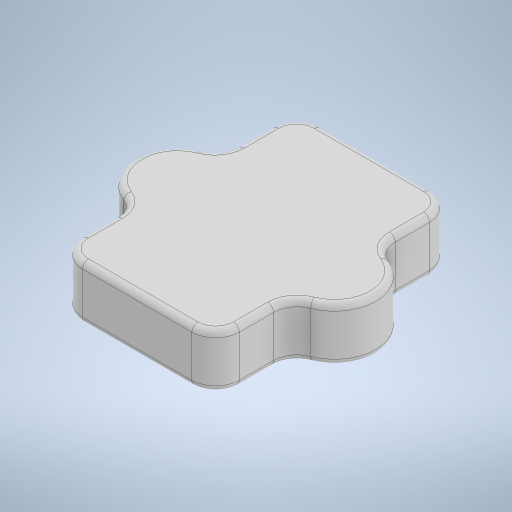
# Autodesk Inventor part: FuselageLock
Saved by Autodesk Inventor 2023 (Build 270158000, 158)
## iProperties
Created: 2023-11-15
Part Number: FuselageLock
Material: Generic
Document SubType Name: Modeling
Designer: Eric
Density: 1 g/cm^3
Appearance: Default
Author: Eric
Autodesk Inventor part; units mm, degrees
ref_plane "YZ Plane" through (0, 0, 0) normal (1, 0, 0) x (0, 1, 0)
ref_plane "XZ Plane" through (0, 0, 0) normal (0, 1, 0) x (-1, 0, 0)
ref_plane "XY Plane" through (0, 0, 0) normal (0, 0, 1) x (1, 0, 0)
sketch "Sketch1" plane through (0, 0, 0) normal (0, 1, 0) x (-1, 0, 0)
  line L0 (6.6, -10) -> (-6.6, -10)
  line L1 (-6.6, -10) -> (-6.6, 10)
  line L2 (-6.6, 10) -> (6.6, 10)
  line L3 (6.6, 10) -> (6.6, -10)
  point P0 (0, 0)
  point P1 (0, -10)
  point P2 (-6.6, 0)
  dimension "d0" = 13.2
  dimension "d1" = 20
  constraints: 8 end point, 2 midpoint, 2 parallel, 1 horizontal, 1 horizontal alignment, 1 perpendicular, 1 vertical alignment
  measures "d0" distance of L0.start L0.end
  measures "d1" distance of L0.end L1.end
extrude "Extrusion1" add sketch "Sketch1" along normal blind 4.5
sketch "Sketch2" plane through (0, 0, 0) normal (0, -1, 0) x (1, 0, 0)
  line L0 (6.6, 10) -> (6.6, -10) projected
  circle A0 centre (6.6, 0) radius 2
  line L1 (-6.6, -10) -> (-6.6, 10) projected
  circle A1 centre (-6.6, 0) radius 2
  circle A2 centre (6.6, 0) radius 3.5
  circle A3 centre (-6.6, 0) radius 3.5
  point P0 (0, 0)
  dimension "d4" = 4
  dimension "d5" = 7
  constraints: 4 centre point, 2 coincident, 2 equal radius, 2 midpoint
  measures "d4" diameter of A0
  measures "d5" diameter of A2
extrude "Extrusion2" add sketch "Sketch2" against normal blind 4.5
extrude "Extrusion3" cut sketch "Sketch2" against normal blind 3 contours A0 L0 | L0 A0 | A1 L1 | L1 A1
fillet "Fillet1" radius 2 8 edges at (6.6, 2.25, -10) (-6.6, 2.25, -10) (6.6, 2.25, 10) (-6.6, 2.25, 10) (6.6, 2.25, -3.5) (6.6, 2.25, 3.5) (-6.6, 2.25, -3.5) (-6.6, 2.25, 3.5)
fillet "Fillet2" radius 0.5 32 edges at (-6.9486, 0, -3.9953) (-6.6, 0, -6.5617) (-6.0142, 0, -9.4142) (0, 0, -10) (6.0142, 0, -9.4142) (6.6, 0, -6.5617) (6.9486, 0, -3.9953) (10.1, 0, 0) (6.9486, 0, 3.9953) (6.6, 0, 6.5617) (6.0142, 0, 9.4142) (0, 0, 10) (-6.0142, 0, 9.4142) (-6.6, 0, 6.5617) (-6.9486, 0, 3.9953) (-10.1, 0, 0) (-6.9486, 4.5, 3.9953) (-6.6, 4.5, 6.5617) (-6.0142, 4.5, 9.4142) (0, 4.5, 10) (6.0142, 4.5, 9.4142) (6.6, 4.5, 6.5617) (6.9486, 4.5, 3.9953) (10.1, 4.5, 0) (6.9486, 4.5, -3.9953) (6.6, 4.5, -6.5617) (6.0142, 4.5, -9.4142) (0, 4.5, -10) (-6.0142, 4.5, -9.4142) (-6.6, 4.5, -6.5617) (-6.9486, 4.5, -3.9953) (-10.1, 4.5, 0)
chamfer "Chamfer1" distance 0.25 angle 45 2 edges at (-8.6, 0, 0) (4.6, 0, 0)
body "Solid1"
